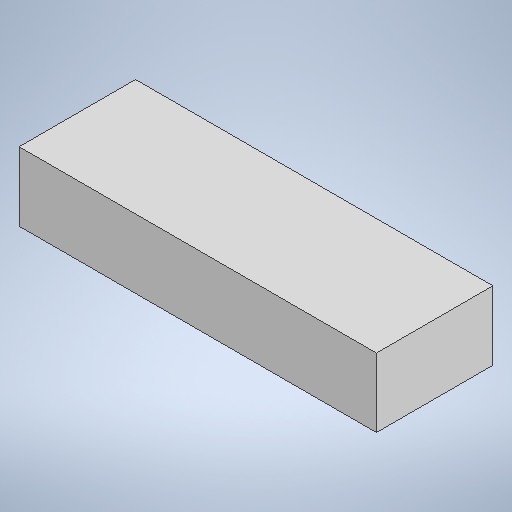
# Autodesk Inventor part: Battery
Saved by Autodesk Inventor 2025 (Build 290162010, 162A)
## iProperties
Created: 2024-09-12
Part Number: Battery
Material: Generic
Document SubType Name: Modeling
Designer: fist5
Density: 1 g/cm^3
Appearance: Default
Author: fist5
Autodesk Inventor part; units mm, degrees
ref_plane "YZ Plane" through (0, 0, 0) normal (1, 0, 0) x (0, 1, 0)
ref_plane "XZ Plane" through (0, 0, 0) normal (0, 1, 0) x (-1, 0, 0)
ref_plane "XY Plane" through (0, 0, 0) normal (0, 0, 1) x (1, 0, 0)
sketch "Sketch1" plane through (0, 0, 0) normal (0, 1, 0) x (-1, 0, 0)
  line L0 (67.5, -22) -> (-67.5, -22)
  line L1 (-67.5, -22) -> (-67.5, 22)
  line L2 (-67.5, 22) -> (67.5, 22)
  line L3 (67.5, 22) -> (67.5, -22)
  line L4 (67.5, -22) -> (-67.5, 22) construction
  line L5 (-67.5, -22) -> (67.5, 22) construction
  point P0 (0, 0)
  dimension "d0" = 135
  dimension "d1" = 44
  constraints: 12 end point, 2 midpoint, 2 parallel, 1 horizontal, 1 perpendicular
  measures "d0" distance between parallel lines of L1 L3
  measures "d1" distance between parallel lines of L2 L0
extrude "Extrusion1" add sketch "Sketch1" along normal blind 26
body "Solid1"
